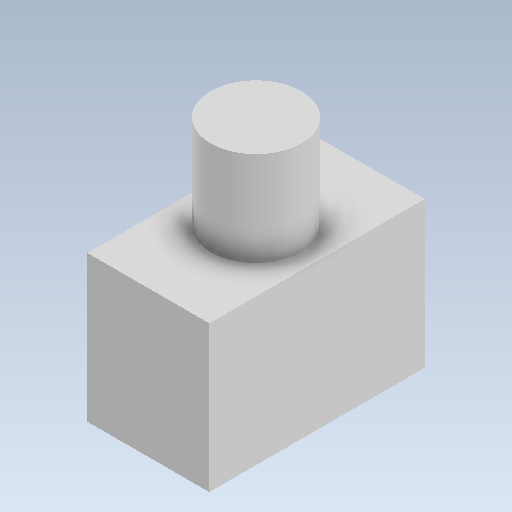
# Autodesk Inventor part: Toggle_Switch
Saved by Autodesk Inventor 2020 (Build 240168000, 168)
## iProperties
Created: 2020-08-08
Part Number: Toggle_Switch
Material: Generic
Document SubType Name: Modeling
Designer: reide
Density: 1 g/cm^3
Appearance: Default
Author: reide
Autodesk Inventor part; units mm, degrees
ref_plane "YZ Plane" through (0, 0, 0) normal (1, 0, 0) x (0, 1, 0)
ref_plane "XZ Plane" through (0, 0, 0) normal (0, 1, 0) x (-1, 0, 0)
ref_plane "XY Plane" through (0, 0, 0) normal (0, 0, 1) x (1, 0, 0)
sketch "Sketch1" plane through (0, 0, 0) normal (0, 1, 0) x (-1, 0, 0)
  line L0 (0, 0) -> (15.85, 0)
  line L1 (15.85, 0) -> (15.85, -28)
  line L2 (15.85, -28) -> (0, -28)
  line L3 (0, -28) -> (0, 0)
  dimension "d0" = 15.85
  dimension "d1" = 28
  constraints: 8 end point, 2 parallel, 1 horizontal, 1 perpendicular
  measures "d0" distance of L1.end L2.end
  measures "d1" distance of L0.end L1.end
extrude "Extrusion1" add sketch "Sketch1" along normal blind 19
sketch "Sketch2" plane through (0, 19, 0) normal (0, 1, 0) x (1, 0, 0)
  line L0 (-15.85, 28) -> (-15.85, 0) projected
  line L1 (-15.85, 0) -> (0, 0) projected
  circle A0 centre (-7.925, 14) radius 5.9
  point P0 (-15.85, 14)
  point P1 (-7.925, 0)
  dimension "d4" = 11.8
  constraints: 2 midpoint, 1 centre point
  measures "d4" diameter of A0
extrude "Extrusion2" add sketch "Sketch2" along normal blind 12.25
body "Solid1"
